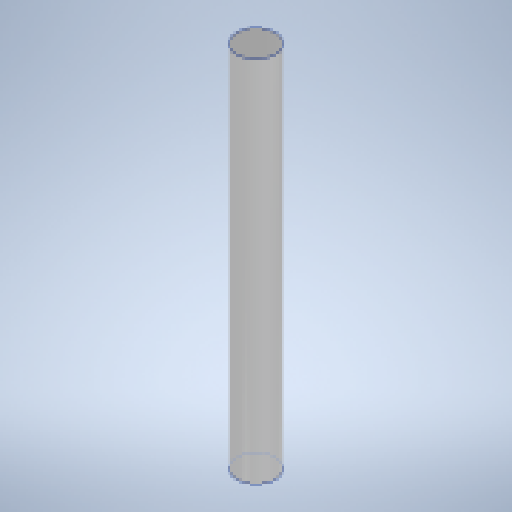
# Autodesk Inventor part: Ф8x77
Saved by Autodesk Inventor 2025 (Build 290162000, 162)
## iProperties
Created: 2025-03-05
Part Number: Ф8x77
Material: アルミニウム 6061
Document SubType Name: Modeling
Designer: Zhopa
Density: 2.7 g/cm^3
Appearance: アルミニウム - フラット
Mass: 10.4502 g
Surface Area: 20.3575 cm^2
Volume: 3.87044 cm^3
Author: Zhopa
Autodesk Inventor part; units mm, degrees
ref_plane "YZ Plane" through (0, 0, 0) normal (1, 0, 0) x (0, 1, 0)
ref_plane "XZ Plane" through (0, 0, 0) normal (0, 1, 0) x (-1, 0, 0)
ref_plane "XY Plane" through (0, 0, 0) normal (0, 0, 1) x (1, 0, 0)
sketch "Sketch1" plane through (0, 0, 0) normal (0, 1, 0) x (-1, 0, 0)
  circle A0 centre (0, 0) radius 4
  dimension "d0" = 8
  constraints: 1 centre point, 1 coincident
  measures "d0" diameter of A0
extrude "Extrusion1" add sketch "Sketch1" along normal blind 77
body "Solid1"
